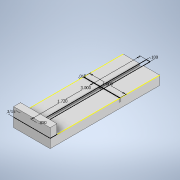
# Autodesk Inventor part: Capillary Cutting Fixture for O-ring system
Saved by Autodesk Inventor 2020 (Build 240168000, 168)
## iProperties
Created: 2022-11-22
Part Number: Capillary Cutting Fixture for O-ring system
Material: Generic
Document SubType Name: Modeling
Designer: Beaucage
Density: 1 g/cm^3
Appearance: Default
Author: Beaucage
Autodesk Inventor part; units mm, degrees
ref_plane "YZ Plane" through (0, 0, 0) normal (1, 0, 0) x (0, 1, 0)
ref_plane "XZ Plane" through (0, 0, 0) normal (0, 1, 0) x (-1, 0, 0)
ref_plane "XY Plane" through (0, 0, 0) normal (0, 0, 1) x (1, 0, 0)
sketch "Sketch1" plane through (0, 0, 0) normal (0, 1, 0) x (-1, 0, 0)
  line L0 (0, 0) -> (25.4, 0)
  line L1 (25.4, 0) -> (25.4, -76.2)
  line L2 (25.4, -76.2) -> (0, -76.2)
  line L3 (0, -76.2) -> (0, 0)
  dimension "d0" = 25.4
  dimension "d1" = 76.2
  constraints: 8 end point, 2 parallel, 1 horizontal, 1 perpendicular
  measures "d0" distance of L1.end L2.end
  measures "d1" distance of L0.end L1.end
extrude "Extrusion1" add sketch "Sketch1" along normal blind 6.35
sketch "Sketch2" plane through (0, 6.35, 0) normal (0, 1, 0) x (1, 0, 0)
  line L0 (-25.4, 0) -> (0, 0) projected
  line L1 (-25.4, 76.2) -> (-25.4, 0) projected
  line L2 (0, 0) -> (-25.4, 0)
  line L3 (-25.4, 0) -> (-25.4, 4.7625)
  line L4 (-25.4, 4.7625) -> (0, 4.7625)
  line L5 (0, 4.7625) -> (0, 0)
  line L6 (-12.7, 4.7625) -> (-11.43, 4.7625)
  line L7 (-11.43, 4.7625) -> (-13.97, 4.7625)
  line L8 (-13.97, 4.7625) -> (-13.97, 80.9625)
  line L9 (-13.97, 80.9625) -> (-11.43, 80.9625)
  line L10 (-11.43, 80.9625) -> (-11.43, 4.7625)
  line L11 (-13.97, 4.7625) -> (-13.97, 48.4505)
  line L12 (-13.97, 48.4505) -> (0, 48.4505)
  line L13 (0, 0) -> (0, 76.2) projected
  line L14 (0, 48.4505) -> (-25.4, 48.4505)
  line L15 (-25.4, 48.4505) -> (-25.4, 48.7045)
  line L16 (-25.4, 48.7045) -> (0, 48.7045)
  line L17 (0, 48.7045) -> (0, 48.4505)
  point P0 (-11.43, 48.4505)
  point P1 (0, 48.7045)
  point P2 (-13.97, 48.7045)
  point P3 (-11.43, 48.7045)
  dimension "d4" = 4.7625
  dimension "d5" = 1.27
  dimension "d6" = 2.54
  dimension "d7" = 76.2
  dimension "d8" = 43.688
  dimension "d9" = 25.4
  dimension "d10" = 0.254
  constraints: 30 end point, 6 parallel, 4 perpendicular, 4 point on line, 3 horizontal, 1 midpoint
  measures "d4" distance of L2.end L3.end
  measures "d5" distance of L6.start L6.end
  measures "d6" distance of L8.end L9.end
  measures "d7" distance of L7.end L8.end
  measures "d8" distance of L7.end L11.end
  measures "d9" distance of L15.end L16.end
  measures "d10" distance of L14.end L15.end
extrude "Extrusion2" add sketch "Sketch2" along normal blind 6.35 contours L1 L4 L5 L0
extrude "Extrusion3" cut sketch "Sketch2" against normal blind 1.27 contours L8 L12 L10 L4 | L8 L16 L10 L12 | L8 L9 L10 L16
extrude "Extrusion4" cut sketch "Sketch2" against normal blind 2.54 contours L1 L16 L8 L14 | L12 L10 L16 L13 | L8 L16 L10 L12
body "Solid1"
